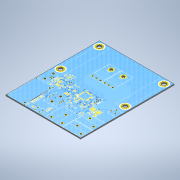
# Autodesk Inventor part: ElectronicLoad_PCB
Saved by Autodesk Inventor 2021 (Build 250183000, 183)
## iProperties
Created: 2020-02-06
Part Number: ElectronicLoad_PCB
Material: Epoxy Resin
Document SubType Name: Modeling
Designer: Bradley
Density: 1.14 g/cm^3
Appearance: Smooth - Medium Gray
Author: Bradley
Autodesk Inventor part; units mm, degrees
ref_plane "YZ Plane" through (0, 0, 0) normal (1, 0, 0) x (0, 1, 0)
ref_plane "XZ Plane" through (0, 0, 0) normal (0, 1, 0) x (-1, 0, 0)
ref_plane "XY Plane" through (0, 0, 0) normal (0, 0, 1) x (1, 0, 0)
sketch "Sketch1" plane through (0, 0, 0) normal (0, 0, 1) x (1, 0, 0)
  line L0 (-52, -65) -> (52, -65)
  line L1 (52, -65) -> (52, 65)
  line L2 (52, 65) -> (-52, 65)
  line L3 (-52, 65) -> (-52, -65)
  line L4 (-52, -65) -> (52, 65) construction
  line L5 (52, -65) -> (-52, 65) construction
  point P0 (0, 0)
  dimension "d0" = 104
  dimension "d1" = 130
  constraints: 12 end point, 2 midpoint, 2 parallel, 1 horizontal, 1 perpendicular
  measures "d0" distance of L2.end L1.end
  measures "d1" distance of L0.end L1.end
extrude "Extrusion1" add sketch "Sketch1" along normal mid plane 1.6
sketch "Sketch2" plane through (0, 0, 0.8) normal (0, 0, 1) x (1, 0, 0)
  line L0 (-52, 65) -> (-52, -65) projected
  line L1 (52, -65) -> (52, 65) projected
  line L2 (-52, 65) -> (52, 65) construction
  line L3 (52, 65) -> (52, -65) construction
  line L4 (52, -65) -> (-52, -65) construction
  line L5 (-52, -65) -> (-52, 65) construction
  point P0 (0, 0)
  point P1 (-52, 0)
  point P2 (-52, 0)
  point P3 (-52, 0)
  point P4 (-52, 0)
  point P5 (-52, 0)
  constraints: 6 midpoint, 2 collinear, 2 other
decal "Decal1"
sketch "Sketch3" plane through (0, 0, -0.8) normal (0, 0, -1) x (-1, 0, 0)
  line L0 (-52, 65) -> (-52, -65) projected
  line L1 (52, -65) -> (52, 65) projected
  line L2 (-52, 65) -> (52, 65) construction
  line L3 (52, 65) -> (52, -65) construction
  line L4 (52, -65) -> (-52, -65) construction
  line L5 (-52, -65) -> (-52, 65) construction
  point P0 (0, 0)
  point P1 (52, 0)
  point P2 (52, 0)
  point P3 (52, 0)
  point P4 (52, 0)
  point P5 (52, 0)
  constraints: 6 midpoint, 2 collinear, 2 other
decal "Decal2"
sketch "Sketch4" plane through (0, 0, 0.8) normal (0, 0, 1) x (1, 0, 0)
  point P0 (0, 0)
  point P1 (45, 58)
  point P2 (45, 4)
  point P3 (-45, 4)
  point P4 (-45, 58)
  constraints: 5 other
hole "Hole1" at (45, 58, 0.8) at (45, 4, 0.8) at (-45, 4, 0.8) at (-45, 58, 0.8) direction (0, 0, -1) diameter 5.7 end through all
sketch "Sketch5" plane through (0, 0, 0.8) normal (0, 0, 1) x (1, 0, 0)
  point P0 (0, 0)
  point P1 (8, 38.5)
  point P2 (-9, 38.5)
  constraints: 3 other
hole "Hole2" at (8, 38.5, 0.8) at (-9, 38.5, 0.8) direction (0, 0, -1) diameter 3.7 end through all
sketch "Sketch19" plane through (0, 0, 0.8) normal (0, 0, 1) x (1, 0, 0)
  point P0 (0, 0)
  point P1 (-12, -41.05)
  point P2 (-12, -28.98)
  constraints: 3 other
hole "Hole16" at (-12, -41.05, 0.8) at (-12, -28.98, 0.8) direction (0, 0, -1) diameter 2.5 end through all
sketch "Sketch20" plane through (0, 0, 0.8) normal (0, 0, 1) x (1, 0, 0)
  point P0 (0, 0)
  point P1 (-44.5, -6.48)
  point P2 (-44.5, -18.52)
  constraints: 3 other
hole "Hole17" at (-44.5, -6.48, 0.8) at (-44.5, -18.52, 0.8) direction (0, 0, -1) diameter 2.3 end through all
sketch "Sketch21" plane through (0, 0, 0.8) normal (0, 0, 1) x (1, 0, 0)
  point P0 (0, 0)
  point P1 (21.35, -60)
  point P2 (47.5, -42.5)
  point P3 (13.85, -47.5)
  point P4 (35, -35)
  point P5 (47.35, -60)
  point P6 (34.85, -52.5)
  point P7 (6.35, -60)
  constraints: 8 other
hole "Hole18" at (21.35, -60, 0.8) at (47.5, -42.5, 0.8) at (13.85, -47.5, 0.8) at (35, -35, 0.8) at (47.35, -60, 0.8) at (34.85, -52.5, 0.8) at (6.35, -60, 0.8) direction (0, 0, -1) diameter 2 end through all
sketch "Sketch22" plane through (0, 0, 0.8) normal (0, 0, 1) x (1, 0, 0)
  point P0 (0, 0)
  point P1 (8, 18)
  point P2 (2.54, 18)
  point P3 (13.46, 18)
  point P4 (-9, 18)
  point P5 (-29.55, -26.45)
  point P6 (-29.55, -61.05)
  point P7 (-14.46, 18)
  point P8 (-3.54, 18)
  constraints: 9 other
hole "Hole19" at (8, 18, 0.8) at (2.54, 18, 0.8) at (13.46, 18, 0.8) at (-9, 18, 0.8) at (-29.55, -26.45, 0.8) at (-29.55, -61.05, 0.8) at (-14.46, 18, 0.8) at (-3.54, 18, 0.8) direction (0, 0, -1) diameter 1.5 end through all
sketch "Sketch23" plane through (0, 0, 0.8) normal (0, 0, 1) x (1, 0, 0)
  point P0 (0, 0)
  point P1 (17.69, -7.95)
  constraints: 2 other
hole "Hole20" at (17.69, -7.95, 0.8) direction (0, 0, -1) diameter 1.25 end through all
sketch "Sketch24" plane through (0, 0, 0.8) normal (0, 0, 1) x (1, 0, 0)
  point P0 (0, 0)
  point P1 (43.5, -6.5)
  point P2 (46.5, -11.2)
  point P3 (40.5, -11.2)
  constraints: 4 other
hole "Hole21" at (43.5, -6.5, 0.8) at (46.5, -11.2, 0.8) at (40.5, -11.2, 0.8) direction (0, 0, -1) diameter 1.2 end through all
sketch "Sketch25" plane through (0, 0, 0.8) normal (0, 0, 1) x (1, 0, 0)
  point P0 (0, 0)
  point P1 (-14.25, -62.5)
  point P2 (-7.75, -62.5)
  point P3 (-7.75, -58)
  point P4 (-21, -8)
  point P5 (-21, -5)
  point P6 (-4.5, -37.5)
  point P7 (19.85, -7.95)
  point P8 (19.85, -10.49)
  point P9 (19.85, -13.03)
  point P10 (19.85, -5.41)
  point P11 (-19, -37.5)
  point P12 (-19, -32.5)
  point P13 (-4.5, -32.5)
  point P14 (-4.5, -35)
  point P15 (-14.25, -58)
  constraints: 16 other
hole "Hole22" at (-14.25, -62.5, 0.8) at (-7.75, -62.5, 0.8) at (-7.75, -58, 0.8) at (-21, -8, 0.8) at (-21, -5, 0.8) at (-4.5, -37.5, 0.8) at (19.85, -7.95, 0.8) at (19.85, -10.49, 0.8) at (19.85, -13.03, 0.8) at (19.85, -5.41, 0.8) at (-19, -37.5, 0.8) at (-19, -32.5, 0.8) at (-4.5, -32.5, 0.8) at (-4.5, -35, 0.8) at (-14.25, -58, 0.8) direction (0, 0, -1) diameter 1 end through all
sketch "Sketch26" plane through (0, 0, 0.8) normal (0, 0, 1) x (1, 0, 0)
  point P0 (0, 0)
  point P1 (-39.79, -13.75)
  point P2 (-39.79, -11.25)
  point P3 (-41.79, -13.75)
  point P4 (-41.79, -11.25)
  constraints: 5 other
hole "Hole23" at (-39.79, -13.75, 0.8) at (-39.79, -11.25, 0.8) at (-41.79, -13.75, 0.8) at (-41.79, -11.25, 0.8) direction (0, 0, -1) diameter 0.9 end through all
sketch "Sketch27" plane through (0, 0, 0.8) normal (0, 0, 1) x (1, 0, 0)
  point P0 (0, 0)
  point P1 (-50.7, -63.85)
  point P2 (-50.7, -23.65)
  point P3 (-27.6, -23.65)
  point P4 (-27.6, -63.85)
  constraints: 5 other
hole "Hole24" at (-50.7, -63.85, 0.8) at (-50.7, -23.65, 0.8) at (-27.6, -23.65, 0.8) at (-27.6, -63.85, 0.8) direction (0, 0, -1) diameter 0.8 end through all
sketch "Sketch28" plane through (0, 0, 0.8) normal (0, 0, 1) x (1, 0, 0)
  point P0 (0, 0)
  point P1 (-27.75, -55.75)
  point P2 (-27.75, -52.75)
  point P3 (-27.75, -54.25)
  point P4 (-27.75, -51.25)
  point P5 (-27.75, -49.75)
  point P6 (-27.75, -34.75)
  point P7 (-27.75, -36.25)
  point P8 (-27.75, -37.75)
  point P9 (-27.75, -46.75)
  point P10 (-27.75, -31.75)
  point P11 (-27.75, -39.25)
  point P12 (-27.75, -40.75)
  point P13 (-27.75, -42.25)
  point P14 (-27.75, -43.75)
  point P15 (-27.75, -45.25)
  point P16 (-27.75, -48.25)
  point P17 (-27.75, -33.25)
  constraints: 18 other
hole "Hole25" at (-27.75, -55.75, 0.8) at (-27.75, -52.75, 0.8) at (-27.75, -54.25, 0.8) at (-27.75, -51.25, 0.8) at (-27.75, -49.75, 0.8) at (-27.75, -34.75, 0.8) at (-27.75, -36.25, 0.8) at (-27.75, -37.75, 0.8) at (-27.75, -46.75, 0.8) at (-27.75, -31.75, 0.8) at (-27.75, -39.25, 0.8) at (-27.75, -40.75, 0.8) at (-27.75, -42.25, 0.8) at (-27.75, -43.75, 0.8) at (-27.75, -45.25, 0.8) at (-27.75, -48.25, 0.8) at (-27.75, -33.25, 0.8) direction (0, 0, -1) diameter 0.6 end through all
sketch "Sketch29" plane through (0, 0, 0.8) normal (0, 0, 1) x (1, 0, 0)
  point P0 (0, 0)
  point P1 (9.135, -23.632)
  point P2 (-20.53, -40.07)
  point P3 (9.597, -24.315)
  point P4 (-20.5, -40.88)
  point P5 (-17.985, -57.181)
  point P6 (-3.35, -41.05)
  point P7 (10.951, -4.053)
  point P8 (-2.4, -26.05)
  point P9 (6.129, -4.053)
  point P10 (-2.3, -17.932)
  point P11 (-7.85, -25.3)
  point P12 (-7.343, -31.193)
  point P13 (5.061, -4.511)
  point P14 (-11.506, -18.641)
  point P15 (-16.5, -27.55)
  point P16 (-14.575, -33.792)
  point P17 (-16.15, -29.45)
  point P18 (6.95, -20.75)
  point P19 (18.4, -17.989)
  point P20 (18.45, -18.799)
  point P21 (13.866, -19.266)
  point P22 (9.001, -27.426)
  point P23 (10.885, -24.715)
  point P24 (15.25, -6.65)
  point P25 (13.7, -11.95)
  point P26 (-35.95, -15)
  point P27 (-36, -6.8)
  point P28 (-34.95, -4.1)
  point P29 (-31.3, -3.7)
  point P30 (14.35, -22.7)
  point P31 (15.65, -23)
  point P32 (15.593, -14.607)
  point P33 (17.792, -12.092)
  point P34 (19.473, -38.385)
  point P35 (18.4, -27.35)
  point P36 (14.6, -3.45)
  point P37 (15.377, -5.123)
  point P38 (14.525, -5.925)
  point P39 (20.3, -38.385)
  point P40 (2.52, -3.8)
  point P41 (4.4, -3.468)
  point P42 (-19.75, -19.65)
  point P43 (-15.861, -14.361)
  point P44 (-28.1, -7.68)
  point P45 (-23.839, -4.412)
  point P46 (-18.8, -6)
  point P47 (-17.75, -8.3)
  point P48 (15.545, -21.85)
  point P49 (13.215, -22.05)
  point P50 (-6.615, -17.3)
  point P51 (-8.55, -17.15)
  point P52 (-6.839, -15.311)
  point P53 (-11.077, -12.427)
  point P54 (-12.53, -12.63)
  point P55 (-0.415, -18.5)
  point P56 (-3.38, -20.72)
  point P57 (11.765, -17.05)
  point P58 (17.036, -17.629)
  point P59 (20.05, -34.21)
  point P60 (19.757, -26.943)
  point P61 (20.45, -18.8)
  point P62 (24.285, -29.563)
  point P63 (20.7, -23.05)
  point P64 (19.814, -21.336)
  point P65 (20.536, -20.914)
  point P66 (-24.8, -17.9)
  point P67 (-36.7, -17.935)
  point P68 (-19.926, -8.884)
  point P69 (-32.35, -14.7)
  point P70 (-32.25, -8.85)
  point P71 (-22.9, -12.95)
  point P72 (-24, -11.6)
  point P73 (-22.25, -12.05)
  point P74 (-25.35, -6.75)
  point P75 (-18.65, -4.1)
  point P76 (-19.698, -18.398)
  point P77 (-16.45, -13.4)
  point P78 (-17.25, -17.4)
  point P79 (-31.05, -8.265)
  point P80 (-9.065, -9.469)
  point P81 (-25.65, -7.53)
  point P82 (-24.315, -8.847)
  point P83 (-21.95, -18)
  point P84 (-2.1, -50.95)
  point P85 (8.65, -26.123)
  point P86 (-20.639, -57.161)
  point P87 (-27.002, -13.775)
  point P88 (-31.37, -17.13)
  point P89 (-7.9, -4.4)
  point P90 (22.873, -13.923)
  point P91 (-1, -19.35)
  point P92 (10.889, -35.861)
  point P93 (8.945, -36.95)
  point P94 (6.15, -35.9)
  point P95 (5.05, -33.95)
  point P96 (16, -19.95)
  point P97 (-31.745, -7.305)
  point P98 (-30.1, -7.335)
  point P99 (12.986, -16.836)
  point P100 (-22.975, -33.55)
  point P101 (-14.215, -44.25)
  point P102 (-21.2, -44.35)
  point P103 (-14.215, -35.2)
  point P104 (-21.05, -35.45)
  point P105 (1.425, -4.4)
  point P106 (16.8, -15.859)
  point P107 (-22.4, -6.4)
  point P108 (16.35, -7.51)
  point P109 (-23.95, 0)
  point P110 (-8.55, -10.1)
  point P111 (-3.05, -4.665)
  point P112 (-2.8, -5.95)
  point P113 (-29.29, -7.335)
  point P114 (-7, -9.45)
  point P115 (-5.589, -11.411)
  point P116 (3.33, -4.053)
  point P117 (7.5, -30.35)
  point P118 (11.8, -18.85)
  point P119 (-7.2, -21.015)
  point P120 (-6.129, -23.479)
  point P121 (-4.961, -18.334)
  point P122 (-3.646, -27.934)
  point P123 (-10.921, -17.229)
  point P124 (-11.506, -17.814)
  point P125 (-3.85, -3.8)
  point P126 (4.308, -18.517)
  point P127 (-11.15, -23.85)
  point P128 (-22.75, -27.35)
  point P129 (-3.26, -12.24)
  point P130 (9.135, -21.15)
  point P131 (1.3, -26.7)
  point P132 (9.135, -21.977)
  point P133 (1.15, -28.3)
  point P134 (-3.15, -27.285)
  point P135 (-7, -23.9)
  point P136 (30.35, -18.85)
  point P137 (23.05, -3.65)
  point P138 (16.118, -3.45)
  point P139 (16.8, -15)
  point P140 (30.848, -18.202)
  point P141 (23.554, -1.796)
  point P142 (12.625, -4.025)
  point P143 (-41.1, 58)
  point P144 (-41.335, 59.334)
  point P145 (-42.012, 60.507)
  point P146 (-43.05, 61.377)
  point P147 (-44.323, 61.841)
  point P148 (9.5, -4.494)
  point P149 (-46.95, 61.377)
  point P150 (-47.988, 60.507)
  point P151 (-48.665, 59.334)
  point P152 (-48.9, 58)
  point P153 (-48.665, 56.666)
  point P154 (-47.988, 55.493)
  point P155 (-46.95, 54.622)
  point P156 (-45.677, 54.159)
  point P157 (-44.323, 54.159)
  point P158 (-43.05, 54.622)
  point P159 (-42.012, 55.493)
  point P160 (-41.335, 56.666)
  point P161 (12, -13.115)
  point P162 (-41.1, 4)
  point P163 (-41.335, 5.334)
  point P164 (-42.012, 6.507)
  point P165 (-43.05, 7.377)
  point P166 (-44.323, 7.841)
  point P167 (-45.677, 7.841)
  point P168 (-46.95, 7.377)
  point P169 (-47.988, 6.507)
  point P170 (-48.665, 5.334)
  point P171 (-48.9, 4)
  point P172 (-48.665, 2.666)
  point P173 (-47.988, 1.493)
  point P174 (-46.95, 0.623)
  point P175 (-45.677, 0.159)
  point P176 (-44.323, 0.159)
  point P177 (-43.05, 0.623)
  point P178 (-42.012, 1.493)
  point P179 (-41.335, 2.666)
  point P180 (-22.7, -36.9)
  point P181 (48.9, 4)
  point P182 (48.665, 5.334)
  point P183 (47.988, 6.507)
  point P184 (-45.677, 61.841)
  point P185 (45.677, 7.841)
  point P186 (44.323, 7.841)
  point P187 (43.05, 7.377)
  point P188 (42.012, 6.507)
  point P189 (41.335, 5.334)
  point P190 (41.1, 4)
  point P191 (41.335, 2.666)
  point P192 (42.012, 1.493)
  point P193 (43.05, 0.623)
  point P194 (44.323, 0.159)
  point P195 (45.677, 0.159)
  point P196 (46.95, 0.623)
  point P197 (47.988, 1.493)
  point P198 (48.665, 2.666)
  point P199 (12.5, -11.945)
  constraints: 221 other
hole "Hole26" at (9.135, -23.632, 0.8) at (-20.53, -40.07, 0.8) at (9.597, -24.315, 0.8) at (-20.5, -40.88, 0.8) at (-17.985, -57.181, 0.8) at (-3.35, -41.05, 0.8) at (10.951, -4.053, 0.8) at (-2.4, -26.05, 0.8) at (6.129, -4.053, 0.8) at (-2.3, -17.932, 0.8) at (-7.85, -25.3, 0.8) at (-7.343, -31.193, 0.8) at (5.061, -4.511, 0.8) at (-11.506, -18.641, 0.8) at (-16.5, -27.55, 0.8) at (-14.575, -33.792, 0.8) at (-16.15, -29.45, 0.8) at (6.95, -20.75, 0.8) at (18.4, -17.989, 0.8) at (18.45, -18.799, 0.8) at (13.866, -19.266, 0.8) at (9.001, -27.426, 0.8) at (10.885, -24.715, 0.8) at (15.25, -6.65, 0.8) at (13.7, -11.95, 0.8) at (-35.95, -15, 0.8) at (-36, -6.8, 0.8) at (-34.95, -4.1, 0.8) at (-31.3, -3.7, 0.8) at (14.35, -22.7, 0.8) at (15.65, -23, 0.8) at (15.593, -14.607, 0.8) at (17.792, -12.092, 0.8) at (19.473, -38.385, 0.8) at (18.4, -27.35, 0.8) at (14.6, -3.45, 0.8) at (15.377, -5.123, 0.8) at (14.525, -5.925, 0.8) at (20.3, -38.385, 0.8) at (2.52, -3.8, 0.8) at (4.4, -3.468, 0.8) at (-19.75, -19.65, 0.8) at (-15.861, -14.361, 0.8) at (-28.1, -7.68, 0.8) at (-23.839, -4.412, 0.8) at (-18.8, -6, 0.8) at (-17.75, -8.3, 0.8) at (15.545, -21.85, 0.8) at (13.215, -22.05, 0.8) at (-6.615, -17.3, 0.8) direction (0, 0, -1) diameter 0.35 end through all and at (-8.55, -17.15, 0.8) (-6.839, -15.311, 0.8) (-11.077, -12.427, 0.8) (-12.53, -12.63, 0.8) (-0.415, -18.5, 0.8) (-3.38, -20.72, 0.8) (11.765, -17.05, 0.8) (17.036, -17.629, 0.8) (20.05, -34.21, 0.8) (19.757, -26.943, 0.8) (20.45, -18.8, 0.8) (24.285, -29.563, 0.8) (20.7, -23.05, 0.8) (19.814, -21.336, 0.8) (20.536, -20.914, 0.8) (-24.8, -17.9, 0.8) (-36.7, -17.935, 0.8) (-19.926, -8.884, 0.8) (-32.35, -14.7, 0.8) (-32.25, -8.85, 0.8) (-22.9, -12.95, 0.8) (-24, -11.6, 0.8) (-22.25, -12.05, 0.8) (-25.35, -6.75, 0.8) (-18.65, -4.1, 0.8) (-19.698, -18.398, 0.8) (-16.45, -13.4, 0.8) (-17.25, -17.4, 0.8) (-31.05, -8.265, 0.8) (-9.065, -9.469, 0.8) (-25.65, -7.53, 0.8) (-24.315, -8.847, 0.8) (-21.95, -18, 0.8) (-2.1, -50.95, 0.8) (8.65, -26.123, 0.8) (-20.639, -57.161, 0.8) (-27.002, -13.775, 0.8) (-31.37, -17.13, 0.8) (-7.9, -4.4, 0.8) (22.873, -13.923, 0.8) (-1, -19.35, 0.8) (10.889, -35.861, 0.8) (8.945, -36.95, 0.8) (6.15, -35.9, 0.8) (5.05, -33.95, 0.8) (16, -19.95, 0.8) (-31.745, -7.305, 0.8) (-30.1, -7.335, 0.8) (12.986, -16.836, 0.8) (-22.975, -33.55, 0.8) (-14.215, -44.25, 0.8) (-21.2, -44.35, 0.8) (-14.215, -35.2, 0.8) (-21.05, -35.45, 0.8) (1.425, -4.4, 0.8) (16.8, -15.859, 0.8) (-22.4, -6.4, 0.8) (16.35, -7.51, 0.8) (-23.95, 0, 0.8) (-8.55, -10.1, 0.8) (-3.05, -4.665, 0.8) (-2.8, -5.95, 0.8) (-29.29, -7.335, 0.8) (-7, -9.45, 0.8) (-5.589, -11.411, 0.8) (3.33, -4.053, 0.8) (7.5, -30.35, 0.8) (11.8, -18.85, 0.8) (-7.2, -21.015, 0.8) (-6.129, -23.479, 0.8) (-4.961, -18.334, 0.8) (-3.646, -27.934, 0.8) (-10.921, -17.229, 0.8) (-11.506, -17.814, 0.8) (-3.85, -3.8, 0.8) (4.308, -18.517, 0.8) (-11.15, -23.85, 0.8) (-22.75, -27.35, 0.8) (-3.26, -12.24, 0.8) (9.135, -21.15, 0.8) (1.3, -26.7, 0.8) (9.135, -21.977, 0.8) (1.15, -28.3, 0.8) (-3.15, -27.285, 0.8) (-7, -23.9, 0.8) (30.35, -18.85, 0.8) (23.05, -3.65, 0.8) (16.118, -3.45, 0.8) (16.8, -15, 0.8) (30.848, -18.202, 0.8) (23.554, -1.796, 0.8) (12.625, -4.025, 0.8) (-41.1, 58, 0.8) (-41.335, 59.334, 0.8) (-42.012, 60.507, 0.8) (-43.05, 61.377, 0.8) (-44.323, 61.841, 0.8) (9.5, -4.494, 0.8) (-46.95, 61.377, 0.8) (-47.988, 60.507, 0.8) (-48.665, 59.334, 0.8) (-48.9, 58, 0.8) (-48.665, 56.666, 0.8) (-47.988, 55.493, 0.8) (-46.95, 54.622, 0.8) (-45.677, 54.159, 0.8) (-44.323, 54.159, 0.8) (-43.05, 54.622, 0.8) (-42.012, 55.493, 0.8) (-41.335, 56.666, 0.8) (12, -13.115, 0.8) (-41.1, 4, 0.8) (-41.335, 5.334, 0.8) (-42.012, 6.507, 0.8) (-43.05, 7.377, 0.8) (-44.323, 7.841, 0.8) (-45.677, 7.841, 0.8) (-46.95, 7.377, 0.8) (-47.988, 6.507, 0.8) (-48.665, 5.334, 0.8) (-48.9, 4, 0.8) (-48.665, 2.666, 0.8) (-47.988, 1.493, 0.8) (-46.95, 0.623, 0.8) (-45.677, 0.159, 0.8) (-44.323, 0.159, 0.8) (-43.05, 0.623, 0.8) (-42.012, 1.493, 0.8) (-41.335, 2.666, 0.8) (-22.7, -36.9, 0.8) (48.9, 4, 0.8) (48.665, 5.334, 0.8) (47.988, 6.507, 0.8) (-45.677, 61.841, 0.8) (45.677, 7.841, 0.8) (44.323, 7.841, 0.8) (43.05, 7.377, 0.8) (42.012, 6.507, 0.8) (41.335, 5.334, 0.8) (41.1, 4, 0.8) (41.335, 2.666, 0.8) (42.012, 1.493, 0.8) (43.05, 0.623, 0.8) (44.323, 0.159, 0.8) (45.677, 0.159, 0.8) (46.95, 0.623, 0.8) (47.988, 1.493, 0.8) (48.665, 2.666, 0.8) (12.5, -11.945, 0.8) (48.9, 58, 0.8) (48.665, 59.334, 0.8) (47.988, 60.507, 0.8) (46.95, 61.377, 0.8) (45.677, 61.841, 0.8) (44.323, 61.841, 0.8) (43.05, 61.377, 0.8) (42.012, 60.507, 0.8) (41.335, 59.334, 0.8) (41.1, 58, 0.8) (41.335, 56.666, 0.8) (42.012, 55.493, 0.8) (43.05, 54.622, 0.8) (44.323, 54.159, 0.8) (45.677, 54.159, 0.8) (46.95, 54.622, 0.8) (47.988, 55.493, 0.8) (48.665, 56.666, 0.8) (9.152, -22.787, 0.8) (-21, -39.395, 0.8) (46.95, 7.377, 0.8)
sketch "Sketch30" plane through (0, 0, 0.8) normal (0, 0, 1) x (1, 0, 0)
  point P0 (0, 0)
  point P1 (13.965, -9.1)
  point P2 (2, -7.5)
  point P3 (-21.8, -23.6)
  point P4 (-23, -31.5)
  constraints: 5 other
hole "Hole27" at (13.965, -9.1, 0.8) at (2, -7.5, 0.8) at (-21.8, -23.6, 0.8) at (-23, -31.5, 0.8) direction (0, 0, -1) diameter 0.3 end through all
body "Solid1"
